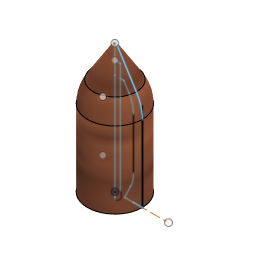
Razzetto v5 (Autodesk Fusion 360 design; units mm, degrees)
Autodesk Fusion 360 part; units mm, degrees
sketch "Schizzo2" plane through (0, 0, 0) normal (0, 1, 0) x (1, 0, 0)
  line L0 (4.25, 0) -> (6.25, 0)
  line L1 (6.25, 0) -> (6.25, -17.4188)
  line L2 (6.25, 0) -> (6.25, -20)
  line L3 (0.2968, -29.5251) -> (4.882, -22.1888)
  line L4 (6.25, 0) -> (4.25, 0)
  line L5 (4.25, -5.8409) -> (4.25, -17.4188)
  line L6 (0, -23) -> (0, -29.6896)
  line L7 (0, 1) -> (0, -23)
  line L8 (4.25, 0) -> (2.25, 0)
  line L9 (2.25, 0) -> (12.25, 0) construction
  line L10 (2.25, 0) -> (3.5942, -2.8825)
  arc A0 (4.25, -5.8409) -> (3.5942, -2.8825) centre (-2.75, -5.8409) ccw
  arc A1 (4.882, -22.1888) -> (6.25, -17.4188) centre (-2.75, -17.4188) ccw
  line L11 (0.9375, -28.5) -> (0, -28.5) construction
  arc A2 (0, -29.6896) -> (0.2968, -29.5251) centre (0, -29.3396) ccw
  line L12 (2.0165, -23) -> (3.186, -21.1288)
  arc A3 (3.186, -21.1288) -> (4.25, -17.4188) centre (-2.75, -17.4188) ccw
  line L13 (4.25, -5.8409) -> (4.25, -17.4188)
  line L14 (1.25, -23) -> (2.0165, -23)
  line L15 (0, -26) -> (1.25, -26)
  line L16 (0, 1) -> (0, 1.5)
  arc A4 (1.25, -0.8292) -> (0, 1.5) centre (0, 0) ccw
  line L17 (1.25, -26) -> (1.25, -0.8292)
  dimension "d9" = 6.25
  dimension "d13" = 20
  dimension "d15" = 2
  dimension "d20" = 2
  dimension "d21" = 65
  dimension "d23" = 7
  dimension "d24" = 9
  dimension "d25" = 0.35
  dimension "d32" = 1.25
  dimension "d33" = 3
  constraint horizontal L0
  constraint perpendicular L0 L1
  constraint perpendicular L0 L2
  constraint perpendicular L1 L4
  constraint perpendicular L0 L5
  constraint perpendicular L5 L8
  constraint horizontal L9
  constraint tangent L5 A0
  constraint tangent L10 A0
  constraint coincident L2.end L3
  constraint tangent L3 A1
  constraint tangent L1 A1
  constraint horizontal L11
  constraint coincident L3 L11.start
  constraint coincident L6 L11.end
  constraint tangent L3 A2
  constraint concentric A1 A3
  constraint tangent L12 A3
  constraint tangent A3 L13
  constraint coincident L6 L15.start
  constraint perpendicular L15 L17
  constraint coincident L14.start L17
  constraint coincident A4.centre origin
  constraint parallel L7 L16
  measures "d9" distance of A4.centre L0.end
  measures "d13" distance of L0.end L2.end
  measures "d15" distance of L0.end L0.start
  measures "d20" distance of L0.start L8.end
  measures "d21" angle of L9 L10
  measures "d23" radius of A0
  measures "d24" radius of A1
  measures "d25" radius of A2
  measures "d32" distance of L15.start L15.end
  measures "d33" diameter of A4
revolve "Rivoluzione5" add sketch "Schizzo2" angle 360 about axis through (0, 0, -1) along (0, 0, 1) contours L0 L1 L2 L3 L4 L5 L6 L8 L10 A0 A1 A2 L12 A3 L13 L14 L15 L17
revolve "Rivoluzione3" [rolled back] along angle 360
ref_plane "Piano di lavoro1" through (0, -3, 0) normal (0, 1, 0) x (0, 0, 1)
revolve "Rivoluzione4" [rolled back] along angle 360
revolve "Rivoluzione2" [suppressed]
sketch "Schizzo3" plane through (0, 0, 0) normal (0, 1, 0) x (1, 0, 0)
  line L0 (0, 1) -> (0, -23)
  constraint vertical L0
revolve "Rivoluzione1" [suppressed]
equation "d9 = ( 12.5 / 2 ) * 1 mm"
named bodies: "razzo", "fiammifero"
